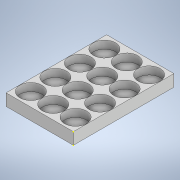
# Autodesk Inventor part: scintillationvialholder2
Saved by Autodesk Inventor 2022 (Build 260153000, 153)
## iProperties
Created: 2022-05-26
Part Number: scintillationvialholder2
Material: Generic
Document SubType Name: Modeling
Designer: Connor
Density: 1 g/cm^3
Appearance: Default
Author: Connor
Autodesk Inventor part; units mm, degrees
ref_plane "YZ Plane" through (0, 0, 0) normal (1, 0, 0) x (0, 1, 0)
ref_plane "XZ Plane" through (0, 0, 0) normal (0, 1, 0) x (-1, 0, 0)
ref_plane "XY Plane" through (0, 0, 0) normal (0, 0, 1) x (1, 0, 0)
sketch "Sketch1" plane through (0, 0, 0) normal (0, 1, 0) x (-1, 0, 0)
  point P0 (0, 0)
sketch "Sketch2" plane through (0, 0, 0) normal (0, 1, 0) x (-1, 0, 0)
  line L0 (0, 0) -> (85.5, 0)
  line L1 (85.5, 0) -> (85.5, -127.8)
  line L2 (85.5, -127.8) -> (0, -127.8)
  line L3 (0, -127.8) -> (0, 0)
  dimension "d0" = 85.5
  dimension "d1" = 127.8
  constraints: 8 end point, 2 parallel, 1 horizontal, 1 perpendicular
  measures "d0" distance of L1.end L2.end
  measures "d1" distance of L0.end L1.end
extrude "Extrusion1" add sketch "Sketch2" along normal blind 15
sketch "Sketch3" plane through (0, 15, 0) normal (0, 1, 0) x (1, 0, 0)
  point P0 (0, 0)
sketch "Sketch5" plane through (0, 15, 0) normal (0, 1, 0) x (1, 0, 0)
  line L0 (0, 127.8) -> (-85.5, 127.8) projected
  line L1 (-85.5, 127.8) -> (-85.5, 0) projected
  line L2 (0, 127.8) -> (-85.5, 127.8)
  line L3 (-85.5, 127.8) -> (-85.5, 124.64)
  line L4 (-85.5, 124.64) -> (0, 124.64)
  line L5 (0, 124.64) -> (0, 127.8)
  line L6 (0, 124.64) -> (-85.5, 124.64)
  line L7 (-85.5, 124.64) -> (-85.5, 96.64)
  line L8 (-85.5, 96.64) -> (0, 96.64)
  line L9 (0, 96.64) -> (0, 124.64)
  line L10 (0, 96.64) -> (-85.5, 96.64)
  line L11 (-85.5, 96.64) -> (-85.5, 93.48)
  line L12 (-85.5, 93.48) -> (0, 93.48)
  line L13 (0, 93.48) -> (0, 96.64)
  line L14 (0, 93.48) -> (-85.5, 93.48)
  line L15 (-85.5, 93.48) -> (-85.5, 65.48)
  line L16 (-85.5, 65.48) -> (0, 65.48)
  line L17 (0, 65.48) -> (0, 93.48)
  line L18 (0, 65.48) -> (-85.5, 65.48)
  line L19 (-85.5, 65.48) -> (-85.5, 62.32)
  line L20 (-85.5, 62.32) -> (0, 62.32)
  line L21 (0, 62.32) -> (0, 65.48)
  line L22 (0, 62.32) -> (-85.5, 62.32)
  line L23 (-85.5, 62.32) -> (-85.5, 34.32)
  line L24 (-85.5, 34.32) -> (0, 34.32)
  line L25 (0, 34.32) -> (0, 62.32)
  line L26 (0, 34.32) -> (-85.5, 34.32)
  line L27 (-85.5, 34.32) -> (-85.5, 31.16)
  line L28 (-85.5, 31.16) -> (0, 31.16)
  line L29 (0, 31.16) -> (0, 34.32)
  line L30 (0, 31.16) -> (-85.5, 31.16)
  line L31 (-85.5, 31.16) -> (-85.5, 3.16)
  line L32 (-85.5, 3.16) -> (0, 3.16)
  line L33 (0, 3.16) -> (0, 31.16)
  line L34 (0, 0) -> (0, 127.8) projected
  line L35 (-85.5, 0) -> (0, 0) projected
  line L36 (0, 127.8) -> (-0.375, 127.8)
  line L37 (-0.375, 127.8) -> (-0.375, 0)
  line L38 (-0.375, 0) -> (0, 0)
  line L39 (0, 0) -> (0, 127.8)
  line L40 (-0.375, 0) -> (-28.375, 0)
  line L41 (-28.375, 0) -> (-28.375, 127.8)
  line L42 (-28.375, 127.8) -> (-0.375, 127.8)
  line L43 (-0.375, 127.8) -> (-0.375, 0)
  line L44 (-28.375, 127.8) -> (-28.75, 127.8)
  line L45 (-28.75, 127.8) -> (-28.75, 3.16)
  line L46 (-28.75, 3.16) -> (-28.375, 3.16)
  line L47 (-28.375, 3.16) -> (-28.375, 127.8)
  line L48 (-28.75, 127.8) -> (-56.75, 127.8)
  line L49 (-56.75, 127.8) -> (-56.75, 3.16)
  line L50 (-56.75, 3.16) -> (-28.75, 3.16)
  line L51 (-28.75, 3.16) -> (-28.75, 127.8)
  line L52 (-56.75, 127.8) -> (-57.125, 127.8)
  line L53 (-57.125, 127.8) -> (-57.125, 3.16)
  line L54 (-57.125, 3.16) -> (-56.75, 3.16)
  line L55 (-56.75, 3.16) -> (-56.75, 127.8)
  line L56 (-57.125, 127.8) -> (-85.125, 127.8)
  line L57 (-85.125, 127.8) -> (-85.125, 3.16)
  line L58 (-85.125, 3.16) -> (-57.125, 3.16)
  line L59 (-57.125, 3.16) -> (-57.125, 127.8)
  circle A0 centre (-14.375, 110.64) radius 14
  circle A1 centre (-14.375, 79.48) radius 14
  circle A2 centre (-14.375, 48.32) radius 14
  circle A3 centre (-14.375, 17.16) radius 14
  circle A4 centre (-42.75, 110.64) radius 14
  circle A5 centre (-42.75, 79.48) radius 14
  circle A6 centre (-42.75, 48.32) radius 14
  circle A7 centre (-42.75, 17.16) radius 14
  circle A8 centre (-71.125, 17.16) radius 14
  circle A9 centre (-71.125, 48.32) radius 14
  circle A10 centre (-71.125, 79.48) radius 14
  circle A11 centre (-71.125, 110.64) radius 14
  dimension "d22" = 3.16
  dimension "d23" = 28
  dimension "d24" = 3.16
  dimension "d25" = 28
  dimension "d26" = 3.16
  dimension "d27" = 28
  dimension "d28" = 3.16
  dimension "d29" = 28
  dimension "d30" = 0.375
  dimension "d31" = 28
  dimension "d32" = 0.375
  dimension "d33" = 28
  dimension "d34" = 0.375
  dimension "d35" = 28
  constraints: 112 end point, 28 parallel, 14 horizontal, 14 perpendicular, 14 point on line, 12 centre point, 7 tangent, 1 other
  measures "d22" distance of L3.end L2.end
  measures "d23" distance of L7.end L6.end
  measures "d24" distance of L11.end L10.end
  measures "d25" distance of L15.end L14.end
  measures "d26" distance of L19.end L18.end
  measures "d27" distance of L23.end L22.end
  measures "d28" distance of L27.end L26.end
  measures "d29" distance of L31.end L30.end
  measures "d30" distance of L38.end L37.end
  measures "d31" distance of L41.end L42.end
  measures "d32" distance of L46.end L45.end
  measures "d33" distance of L50.end L49.end
  measures "d34" distance of L54.end L53.end
  measures "d35" distance of L58.end L57.end
extrude "Extrusion3" cut sketch "Sketch5" against normal blind 10 contours A0 | A4 | A1 | A11 | A2 | A5 | A3 | A10 | A6 | A7 | A9 | A8
body "Solid1"
